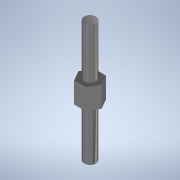
# Autodesk Inventor part: wheel_shock_pin
Saved by Autodesk Inventor 2020 (Build 240168000, 168)
## iProperties
Created: 2016-01-05
Part Number: wheel_shock_pin
Material: Genérico
Document SubType Name: Modeling
Designer: MIGUEL ANGEL
Density: 1 g/cm^3
Appearance: Cromo - Negro Pulido
Author: MIGUEL ANGEL
Autodesk Inventor part; units mm, degrees
ref_plane "YZ Plane" through (0, 0, 0) normal (1, 0, 0) x (0, 1, 0)
ref_plane "XZ Plane" through (0, 0, 0) normal (0, 1, 0) x (-1, 0, 0)
sketch "Boceto1" plane through (0, 0, 0) normal (0, 0, 1) x (1, 0, 0)
  circle A0 centre (0, 0) radius 3
  dimension "d0" = 6
  constraints: 1 centre point, 1 coincident
  measures "d0" diameter of A0
extrude "Extrusión1" add sketch "Boceto1" along normal blind 26
sketch "Boceto2" plane through (0, 0, 26) normal (0, 0, 1) x (1, 0, 0)
  line L0 (6, 0) -> (3, -5.1962)
  line L1 (3, -5.1962) -> (-3, -5.1962)
  line L2 (-3, -5.1962) -> (-6, 0)
  line L3 (-6, 0) -> (-3, 5.1962)
  line L4 (-3, 5.1962) -> (3, 5.1962)
  line L5 (3, 5.1962) -> (6, 0)
  point P0 (0, 0)
  point P1 (0, 0)
  point P2 (0, 5.1962)
  dimension "d3" = 6
  constraints: 12 end point, 1 coincident, 1 midpoint, 1 vertical alignment, 13 other
  measures "d3" distance of L3.end L4.end
extrude "Extrusión2" add sketch "Boceto2" along normal blind 10.75
ref_plane "Plano de trabajo1" through (0, 0, 31.375) normal (0, 0, 1) x (1, 0, 0)
mirror "Simetría1" about plane through (0, 0, 31.375) normal (0, 0, 1) of "Extrusión1"
